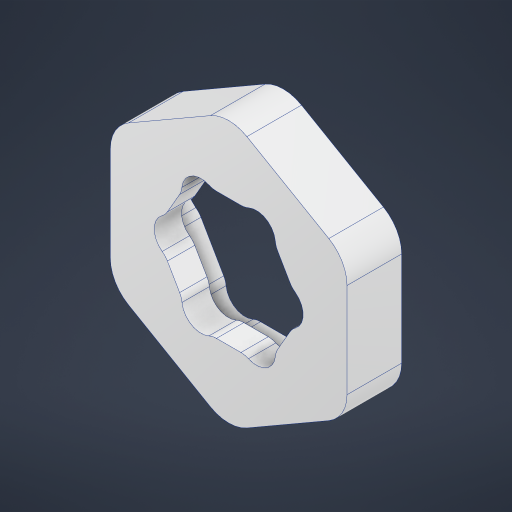
# Autodesk Inventor part: Handmade tiered cover_9mm_Wide_ALU_Cover
Saved by Autodesk Inventor 2024 (Build 280153000, 153)
## iProperties
Created: 2024-06-26
Part Number: Handmade tiered cover_9mm_Wide_ALU_Cover
Material: 알루미늄 6061
Document SubType Name: Sheet Metal
Designer: ASUS
Density: 2.7 g/cm^3
Appearance: 알루미늄 - 평지
Flat Pattern Width: 1.3 cm
Flat Pattern Length: 1.43923 cm
Flat Pattern Area: 1.871 cm^2
Sheet Metal Rule: 기본값
Sheet Metal Width: 13.000 mm
Sheet Metal Length: 14.392 mm
Sheet Metal Area: 187.100 mm^2
Author: ASUS
Autodesk Inventor part; units mm, degrees
ref_plane "YZ Plane" through (0, 0, 0) normal (1, 0, 0) x (0, 1, 0)
ref_plane "XZ Plane" through (0, 0, 0) normal (0, 1, 0) x (-1, 0, 0)
ref_plane "XY Plane" through (0, 0, 0) normal (0, 0, 1) x (1, 0, 0)
sketch "스케치1" plane through (0, 0, 0) normal (0, 0, 1) x (1, 0, 0)
  ellipse E0 centre (98.6441, 1.3888) end of major axis (99.6441, 1.3888) minor radius 1 (99.4578, 1.9701) -> (99.1441, 2.2549) ccw projected
  line L0 (99.1441, 2.2549) -> (97.9803, 2.9268) projected
  ellipse E1 centre (97.4803, 2.0608) end of major axis (98.4803, 2.0608) minor radius 1 (97.9803, 2.9268) -> (97.5768, 3.0561) ccw projected
  ellipse E2 centre (97.6782, 4.1012) end of major axis (96.6282, 4.1012) minor radius 1.05 (96.7225, 4.5359) -> (97.5768, 3.0561) ccw projected
  ellipse E3 centre (95.8122, 4.95) end of major axis (96.8122, 4.95) minor radius 1 (96.7225, 4.5359) -> (96.8122, 4.95) ccw projected
  line L1 (96.8122, 4.95) -> (96.8122, 6.2938) projected
  ellipse E4 centre (95.8122, 6.2938) end of major axis (96.8122, 6.2938) minor radius 1 (96.8122, 6.2938) -> (96.7225, 6.7079) ccw projected
  ellipse E5 centre (97.6782, 7.1426) end of major axis (96.6282, 7.1426) minor radius 1.05 (97.5768, 8.1877) -> (96.7225, 6.7079) ccw projected
  ellipse E6 centre (97.4803, 9.183) end of major axis (96.4803, 9.1831) minor radius 1 (97.5768, 8.1877) -> (97.9803, 8.317) ccw projected
  line L2 (97.9803, 8.317) -> (99.1441, 8.989) projected
  ellipse E7 centre (98.6441, 9.855) end of major axis (97.6441, 9.855) minor radius 1 (99.1441, 8.989) -> (99.4578, 9.2737) ccw projected
  ellipse E8 centre (100.3122, 8.6634) end of major axis (99.2622, 8.6634) minor radius 1.05 (101.1666, 9.2737) -> (99.4578, 9.2737) ccw projected
  ellipse E9 centre (101.9803, 9.855) end of major axis (100.9803, 9.855) minor radius 1 (101.1666, 9.2737) -> (101.4803, 8.989) ccw projected
  line L3 (101.4803, 8.989) -> (102.6441, 8.317) projected
  ellipse E10 centre (103.1441, 9.183) end of major axis (102.1441, 9.1831) minor radius 1 (102.6441, 8.317) -> (103.0476, 8.1877) ccw projected
  ellipse E11 centre (102.9462, 7.1426) end of major axis (101.8962, 7.1426) minor radius 1.05 (103.9019, 6.7079) -> (103.0476, 8.1877) ccw projected
  ellipse E12 centre (104.8122, 6.2938) end of major axis (103.8122, 6.2938) minor radius 1 (103.9019, 6.7079) -> (103.8122, 6.2938) ccw projected
  line L4 (103.8122, 6.2938) -> (103.8122, 4.95) projected
  ellipse E13 centre (104.8122, 4.95) end of major axis (103.8122, 4.95) minor radius 1 (103.8122, 4.95) -> (103.9019, 4.5359) ccw projected
  ellipse E14 centre (102.9462, 4.1012) end of major axis (101.8962, 4.1012) minor radius 1.05 (103.0476, 3.0561) -> (103.9019, 4.5359) ccw projected
  ellipse E15 centre (103.1441, 2.0608) end of major axis (104.1441, 2.0608) minor radius 1 (103.0476, 3.0561) -> (102.6441, 2.9268) ccw projected
  line L5 (102.6441, 2.9268) -> (101.4803, 2.2549) projected
  ellipse E16 centre (101.9803, 1.3888) end of major axis (102.9803, 1.3888) minor radius 1 (101.4803, 2.2549) -> (101.1666, 1.9701) ccw projected
  ellipse E17 centre (100.3122, 2.5805) end of major axis (99.2622, 2.5805) minor radius 1.05 (99.4578, 1.9701) -> (101.1666, 1.9701) ccw projected
  ellipse E18 centre (95.8122, 3.0238) end of major axis (93.8122, 3.0238) minor radius 2 (93.8122, 3.0238) -> (94.8122, 1.2918) ccw projected
  line L6 (94.8122, 1.2918) -> (99.3122, -1.3063) projected
  ellipse E19 centre (100.3122, 0.4258) end of major axis (102.3122, 0.4258) minor radius 2 (99.3122, -1.3063) -> (101.3122, -1.3063) ccw projected
  line L7 (101.3122, -1.3063) -> (105.8122, 1.2918) projected
  ellipse E20 centre (104.8122, 3.0238) end of major axis (106.8122, 3.0238) minor radius 2 (105.8122, 1.2918) -> (106.8122, 3.0238) ccw projected
  line L8 (106.8122, 3.0238) -> (106.8122, 8.22) projected
  ellipse E21 centre (104.8122, 8.22) end of major axis (106.8122, 8.22) minor radius 2 (106.8122, 8.22) -> (105.8122, 9.952) ccw projected
  line L9 (105.8122, 9.952) -> (101.3122, 12.5501) projected
  ellipse E22 centre (100.3122, 10.818) end of major axis (98.3122, 10.8181) minor radius 2 (101.3122, 12.5501) -> (99.3122, 12.5501) ccw projected
  line L10 (99.3122, 12.5501) -> (94.8122, 9.952) projected
  ellipse E23 centre (95.8122, 8.22) end of major axis (97.8122, 8.22) minor radius 2 (94.8122, 9.952) -> (93.8122, 8.22) ccw projected
  line L11 (93.8122, 8.22) -> (93.8122, 3.0238) projected
  line L12 (97.9803, 2.9239) -> (99.1441, 2.252) projected
  ellipse E24 centre (98.6441, 1.386) end of major axis (99.6441, 1.3859) minor radius 1 (99.4578, 1.9672) -> (99.1441, 2.252) ccw projected
  ellipse E25 centre (100.3122, 2.5776) end of major axis (99.2622, 2.5776) minor radius 1.05 (99.4578, 1.9672) -> (101.1666, 1.9672) ccw projected
  ellipse E26 centre (101.9803, 1.386) end of major axis (102.9803, 1.3859) minor radius 1 (101.4803, 2.252) -> (101.1666, 1.9672) ccw projected
  line L13 (101.4803, 2.252) -> (102.6441, 2.9239) projected
  ellipse E27 centre (103.1441, 2.0579) end of major axis (104.1441, 2.0579) minor radius 1 (103.0476, 3.0532) -> (102.6441, 2.9239) ccw projected
  ellipse E28 centre (102.9462, 4.0983) end of major axis (101.8962, 4.0983) minor radius 1.05 (103.0476, 3.0532) -> (103.9019, 4.533) ccw projected
  ellipse E29 centre (104.8122, 4.9471) end of major axis (105.8122, 4.9471) minor radius 1 (103.8122, 4.9471) -> (103.9019, 4.533) ccw projected
  line L14 (103.8122, 4.9471) -> (103.8122, 6.291) projected
  ellipse E30 centre (104.8122, 6.291) end of major axis (105.8122, 6.291) minor radius 1 (103.9019, 6.705) -> (103.8122, 6.291) ccw projected
  ellipse E31 centre (102.9462, 7.1397) end of major axis (101.8962, 7.1398) minor radius 1.05 (103.9019, 6.705) -> (103.0476, 8.1848) ccw projected
  ellipse E32 centre (103.1441, 9.1802) end of major axis (102.1441, 9.1802) minor radius 1 (102.6441, 8.3141) -> (103.0476, 8.1848) ccw projected
  line L15 (102.6441, 8.3141) -> (101.4803, 8.9861) projected
  ellipse E33 centre (101.9803, 9.8521) end of major axis (100.9803, 9.8521) minor radius 1 (101.1666, 9.2708) -> (101.4803, 8.9861) ccw projected
  ellipse E34 centre (100.3122, 8.6605) end of major axis (99.2622, 8.6605) minor radius 1.05 (101.1666, 9.2708) -> (99.4578, 9.2708) ccw projected
  ellipse E35 centre (98.6441, 9.8521) end of major axis (97.6441, 9.8521) minor radius 1 (99.1441, 8.9861) -> (99.4578, 9.2708) ccw projected
  line L16 (99.1441, 8.9861) -> (97.9803, 8.3141) projected
  ellipse E36 centre (97.4803, 9.1802) end of major axis (96.4803, 9.1802) minor radius 1 (97.5768, 8.1848) -> (97.9803, 8.3141) ccw projected
  ellipse E37 centre (97.6782, 7.1397) end of major axis (96.6282, 7.1398) minor radius 1.05 (97.5768, 8.1848) -> (96.7225, 6.705) ccw projected
  ellipse E38 centre (95.8122, 6.291) end of major axis (94.8122, 6.291) minor radius 1 (96.8122, 6.291) -> (96.7225, 6.705) ccw projected
  line L17 (96.8122, 6.291) -> (96.8122, 4.9471) projected
  ellipse E39 centre (95.8122, 4.9471) end of major axis (94.8122, 4.9471) minor radius 1 (96.7225, 4.533) -> (96.8122, 4.9471) ccw projected
  ellipse E40 centre (97.6782, 4.0983) end of major axis (96.6282, 4.0983) minor radius 1.05 (96.7225, 4.533) -> (97.5768, 3.0532) ccw projected
  ellipse E41 centre (97.4803, 2.0579) end of major axis (98.4803, 2.0579) minor radius 1 (97.9803, 2.9239) -> (97.5768, 3.0532) ccw projected
  ellipse E42 centre (100.3122, 5.619) end of major axis (98.1872, 5.619) minor radius 2.125 projected
  ellipse E43 centre (-1.6681, -4.2302) end of major axis (-0.6681, -4.2302) minor radius 1 (-0.8544, -3.6489) -> (-1.1681, -3.3642) ccw
  line L18 (-1.1681, -3.3642) -> (-2.3319, -2.6922)
  ellipse E44 centre (-2.8319, -3.5583) end of major axis (-1.8319, -3.5583) minor radius 1 (-2.3319, -2.6922) -> (-2.7354, -2.5629) ccw
  ellipse E45 centre (-2.634, -1.5178) end of major axis (-3.684, -1.5178) minor radius 1.05 (-3.5897, -1.0831) -> (-2.7354, -2.5629) ccw
  ellipse E46 centre (-4.5, -0.669) end of major axis (-3.5, -0.6691) minor radius 1 (-3.5897, -1.0831) -> (-3.5, -0.669) ccw
  line L19 (-3.5, -0.669) -> (-3.5, 0.6748)
  ellipse E47 centre (-4.5, 0.6748) end of major axis (-3.5, 0.6748) minor radius 1 (-3.5, 0.6748) -> (-3.5897, 1.0889) ccw
  ellipse E48 centre (-2.634, 1.5236) end of major axis (-3.684, 1.5236) minor radius 1.05 (-2.7354, 2.5687) -> (-3.5897, 1.0889) ccw
  ellipse E49 centre (-2.8319, 3.564) end of major axis (-3.8319, 3.564) minor radius 1 (-2.7354, 2.5687) -> (-2.3319, 2.698) ccw
  line L20 (-2.3319, 2.698) -> (-1.1681, 3.3699)
  ellipse E50 centre (-1.6681, 4.236) end of major axis (-2.6681, 4.236) minor radius 1 (-1.1681, 3.3699) -> (-0.8544, 3.6547) ccw
  ellipse E51 centre (0, 3.0443) end of major axis (-1.05, 3.0443) minor radius 1.05 (0.8544, 3.6547) -> (-0.8544, 3.6547) ccw
  ellipse E52 centre (1.6681, 4.236) end of major axis (0.6681, 4.236) minor radius 1 (0.8544, 3.6547) -> (1.1681, 3.3699) ccw
  line L21 (1.1681, 3.3699) -> (2.3319, 2.698)
  ellipse E53 centre (2.8319, 3.564) end of major axis (1.8319, 3.564) minor radius 1 (2.3319, 2.698) -> (2.7354, 2.5687) ccw
  ellipse E54 centre (2.634, 1.5236) end of major axis (1.584, 1.5236) minor radius 1.05 (3.5897, 1.0889) -> (2.7354, 2.5687) ccw
  ellipse E55 centre (4.5, 0.6748) end of major axis (3.5, 0.6748) minor radius 1 (3.5897, 1.0889) -> (3.5, 0.6748) ccw
  line L22 (3.5, 0.6748) -> (3.5, -0.6691)
  ellipse E56 centre (4.5, -0.6691) end of major axis (3.5, -0.669) minor radius 1 (3.5, -0.6691) -> (3.5897, -1.0831) ccw
  ellipse E57 centre (2.634, -1.5178) end of major axis (1.584, -1.5178) minor radius 1.05 (2.7354, -2.5629) -> (3.5897, -1.0831) ccw
  ellipse E58 centre (2.8319, -3.5583) end of major axis (3.8319, -3.5583) minor radius 1 (2.7354, -2.5629) -> (2.3319, -2.6922) ccw
  line L23 (2.3319, -2.6922) -> (1.1681, -3.3642)
  ellipse E59 centre (1.6681, -4.2302) end of major axis (2.6681, -4.2302) minor radius 1 (1.1681, -3.3642) -> (0.8544, -3.6489) ccw
  ellipse E60 centre (0, -3.0386) end of major axis (-1.05, -3.0386) minor radius 1.05 (-0.8544, -3.6489) -> (0.8544, -3.6489) ccw
  ellipse E61 centre (-4.5, -2.5952) end of major axis (-6.5, -2.5952) minor radius 2 (-6.5, -2.5952) -> (-5.5, -4.3272) ccw
  line L24 (-5.5, -4.3272) -> (-1, -6.9253)
  ellipse E62 centre (0, -5.1933) end of major axis (2, -5.1933) minor radius 2 (-1, -6.9253) -> (1, -6.9253) ccw
  line L25 (1, -6.9253) -> (5.5, -4.3272)
  ellipse E63 centre (4.5, -2.5952) end of major axis (6.5, -2.5952) minor radius 2 (5.5, -4.3272) -> (6.5, -2.5952) ccw
  line L26 (6.5, -2.5952) -> (6.5, 2.601)
  ellipse E64 centre (4.5, 2.601) end of major axis (6.5, 2.601) minor radius 2 (6.5, 2.601) -> (5.5, 4.333) ccw
  line L27 (5.5, 4.333) -> (1, 6.9311)
  ellipse E65 centre (0, 5.199) end of major axis (-2, 5.199) minor radius 2 (1, 6.9311) -> (-1, 6.9311) ccw
  line L28 (-1, 6.9311) -> (-5.5, 4.333)
  ellipse E66 centre (-4.5, 2.601) end of major axis (-2.5, 2.6009) minor radius 2 (-5.5, 4.333) -> (-6.5, 2.601) ccw
  line L29 (-6.5, 2.601) -> (-6.5, -2.5952)
  line L30 (-2.3319, -2.6951) -> (-1.1681, -3.367)
  ellipse E67 centre (-1.6681, -4.2331) end of major axis (-0.6681, -4.2331) minor radius 1 (-0.8544, -3.6518) -> (-1.1681, -3.367) ccw
  ellipse E68 centre (0, -3.0414) end of major axis (-1.05, -3.0414) minor radius 1.05 (-0.8544, -3.6518) -> (0.8544, -3.6518) ccw
  ellipse E69 centre (1.6681, -4.2331) end of major axis (2.6681, -4.2331) minor radius 1 (1.1681, -3.367) -> (0.8544, -3.6518) ccw
  line L31 (1.1681, -3.367) -> (2.3319, -2.6951)
  ellipse E70 centre (2.8319, -3.5611) end of major axis (3.8319, -3.5611) minor radius 1 (2.7354, -2.5658) -> (2.3319, -2.6951) ccw
  ellipse E71 centre (2.634, -1.5207) end of major axis (1.584, -1.5207) minor radius 1.05 (2.7354, -2.5658) -> (3.5897, -1.086) ccw
  ellipse E72 centre (4.5, -0.6719) end of major axis (5.5, -0.6719) minor radius 1 (3.5, -0.6719) -> (3.5897, -1.086) ccw
  line L32 (3.5, -0.6719) -> (3.5, 0.6719)
  ellipse E73 centre (4.5, 0.6719) end of major axis (5.5, 0.6719) minor radius 1 (3.5897, 1.086) -> (3.5, 0.6719) ccw
  ellipse E74 centre (2.634, 1.5207) end of major axis (1.584, 1.5207) minor radius 1.05 (3.5897, 1.086) -> (2.7354, 2.5658) ccw
  ellipse E75 centre (2.8319, 3.5611) end of major axis (1.8319, 3.5611) minor radius 1 (2.3319, 2.6951) -> (2.7354, 2.5658) ccw
  line L33 (2.3319, 2.6951) -> (1.1681, 3.367)
  ellipse E76 centre (1.6681, 4.2331) end of major axis (0.6681, 4.2331) minor radius 1 (0.8544, 3.6518) -> (1.1681, 3.367) ccw
  ellipse E77 centre (0, 3.0414) end of major axis (-1.05, 3.0415) minor radius 1.05 (0.8544, 3.6518) -> (-0.8544, 3.6518) ccw
  ellipse E78 centre (-1.6681, 4.2331) end of major axis (-2.6681, 4.2331) minor radius 1 (-1.1681, 3.367) -> (-0.8544, 3.6518) ccw
  line L34 (-1.1681, 3.367) -> (-2.3319, 2.6951)
  ellipse E79 centre (-2.8319, 3.5611) end of major axis (-3.8319, 3.5611) minor radius 1 (-2.7354, 2.5658) -> (-2.3319, 2.6951) ccw
  ellipse E80 centre (-2.634, 1.5207) end of major axis (-3.684, 1.5207) minor radius 1.05 (-2.7354, 2.5658) -> (-3.5897, 1.086) ccw
  ellipse E81 centre (-4.5, 0.6719) end of major axis (-5.5, 0.6719) minor radius 1 (-3.5, 0.6719) -> (-3.5897, 1.086) ccw
  line L35 (-3.5, 0.6719) -> (-3.5, -0.6719)
  ellipse E82 centre (-4.5, -0.6719) end of major axis (-5.5, -0.6719) minor radius 1 (-3.5897, -1.086) -> (-3.5, -0.6719) ccw
  ellipse E83 centre (-2.634, -1.5207) end of major axis (-3.684, -1.5207) minor radius 1.05 (-3.5897, -1.086) -> (-2.7354, -2.5658) ccw
  ellipse E84 centre (-2.8319, -3.5611) end of major axis (-1.8319, -3.5611) minor radius 1 (-2.3319, -2.6951) -> (-2.7354, -2.5658) ccw
  ellipse E85 centre (0, 0) end of major axis (-2.125, 0) minor radius 2.125
  point P0 (-3.684, -1.5193)
  point P1 (-3.684, 1.5222)
  point P2 (3.684, 1.5222)
  point P3 (3.5, 0.6721)
  point P4 (3.684, -1.5193)
  constraints: 36 end point, 213 other
extrude "돌출1" add sketch "스케치1" along normal blind 3 contours L29 E66 L28 E65 L27 E64 L26 E63 L25 E62 L24 E61
sketch "스케치2" plane through (0, 0, 3) normal (0, 0, 1) x (1, 0, 0)
  ellipse E0 centre (-4.5, -2.5952) end of major axis (-6.5, -2.5952) minor radius 2 (-6.5, -2.5952) -> (-5.5, -4.3272) ccw projected
  line L0 (-5.5, -4.3272) -> (-1, -6.9253) projected
  ellipse E1 centre (0, -5.1933) end of major axis (2, -5.1933) minor radius 2 (-1, -6.9253) -> (1, -6.9253) ccw projected
  line L1 (1, -6.9253) -> (5.5, -4.3272) projected
  ellipse E2 centre (4.5, -2.5952) end of major axis (6.5, -2.5952) minor radius 2 (5.5, -4.3272) -> (6.5, -2.5952) ccw projected
  line L2 (6.5, -2.5952) -> (6.5, 2.601) projected
  ellipse E3 centre (4.5, 2.601) end of major axis (6.5, 2.601) minor radius 2 (6.5, 2.601) -> (5.5, 4.333) ccw projected
  line L3 (5.5, 4.333) -> (1, 6.9311) projected
  ellipse E4 centre (0, 5.199) end of major axis (-2, 5.199) minor radius 2 (1, 6.9311) -> (-1, 6.9311) ccw projected
  line L4 (-1, 6.9311) -> (-5.5, 4.333) projected
  ellipse E5 centre (-4.5, 2.601) end of major axis (-2.5, 2.6009) minor radius 2 (-5.5, 4.333) -> (-6.5, 2.601) ccw projected
  line L5 (-6.5, 2.601) -> (-6.5, -2.5952) projected
  ellipse E6 centre (-2.8319, -3.5611) end of major axis (-1.8319, -3.5611) minor radius 1 (-2.3319, -2.6951) -> (-2.7354, -2.5658) ccw projected
  ellipse E7 centre (-2.634, -1.5207) end of major axis (-1.584, -1.5207) minor radius 1.05 (-3.684, -1.5193) -> (-2.7354, -2.5658) ccw projected
  ellipse E8 centre (-2.634, -1.5178) end of major axis (-1.584, -1.5178) minor radius 1.05 (-3.5897, -1.0831) -> (-3.684, -1.5193) ccw projected
  ellipse E9 centre (-4.5, -0.669) end of major axis (-3.5, -0.6691) minor radius 1 (-3.5897, -1.0831) -> (-3.5, -0.669) ccw projected
  line L6 (-3.5, -0.669) -> (-3.5, 0.6748) projected
  ellipse E10 centre (-4.5, 0.6719) end of major axis (-5.5, 0.6719) minor radius 1 (-3.5, 0.6748) -> (-3.5897, 1.086) ccw projected
  ellipse E11 centre (-2.634, 1.5207) end of major axis (-1.584, 1.5207) minor radius 1.05 (-3.684, 1.5222) -> (-3.5897, 1.086) ccw projected
  ellipse E12 centre (-2.634, 1.5236) end of major axis (-1.584, 1.5236) minor radius 1.05 (-2.7354, 2.5687) -> (-3.684, 1.5222) ccw projected
  ellipse E13 centre (-2.8319, 3.564) end of major axis (-3.8319, 3.564) minor radius 1 (-2.7354, 2.5687) -> (-2.3319, 2.698) ccw projected
  line L7 (-2.3319, 2.698) -> (-1.1681, 3.3699) projected
  ellipse E14 centre (-1.6681, 4.236) end of major axis (-2.6681, 4.236) minor radius 1 (-1.1681, 3.3699) -> (-0.8544, 3.6547) ccw projected
  ellipse E15 centre (0, 3.0443) end of major axis (1.05, 3.0443) minor radius 1.05 (0.8544, 3.6547) -> (-0.8544, 3.6547) ccw projected
  ellipse E16 centre (1.6681, 4.236) end of major axis (0.6681, 4.236) minor radius 1 (0.8544, 3.6547) -> (1.1681, 3.3699) ccw projected
  line L8 (1.1681, 3.3699) -> (2.3319, 2.698) projected
  ellipse E17 centre (2.8319, 3.564) end of major axis (1.8319, 3.564) minor radius 1 (2.3319, 2.698) -> (2.7354, 2.5687) ccw projected
  ellipse E18 centre (2.634, 1.5236) end of major axis (3.684, 1.5236) minor radius 1.05 (3.684, 1.5222) -> (2.7354, 2.5687) ccw projected
  ellipse E19 centre (2.634, 1.5207) end of major axis (3.684, 1.5207) minor radius 1.05 (3.5897, 1.086) -> (3.684, 1.5222) ccw projected
  ellipse E20 centre (4.5, 0.6719) end of major axis (5.5, 0.6719) minor radius 1 (3.5897, 1.086) -> (3.5, 0.6721) ccw projected
  line L9 (3.5, 0.6721) -> (3.5, -0.6691) projected
  ellipse E21 centre (4.5, -0.6691) end of major axis (3.5, -0.669) minor radius 1 (3.5, -0.6691) -> (3.5897, -1.0831) ccw projected
  ellipse E22 centre (2.634, -1.5178) end of major axis (3.684, -1.5178) minor radius 1.05 (3.684, -1.5193) -> (3.5897, -1.0831) ccw projected
  ellipse E23 centre (2.634, -1.5207) end of major axis (3.684, -1.5207) minor radius 1.05 (2.7354, -2.5658) -> (3.684, -1.5193) ccw projected
  ellipse E24 centre (2.8319, -3.5611) end of major axis (3.8319, -3.5611) minor radius 1 (2.7354, -2.5658) -> (2.3319, -2.6951) ccw projected
  line L10 (2.3319, -2.6951) -> (1.1681, -3.367) projected
  ellipse E25 centre (1.6681, -4.2331) end of major axis (2.6681, -4.2331) minor radius 1 (1.1681, -3.367) -> (0.8544, -3.6518) ccw projected
  ellipse E26 centre (0, -3.0414) end of major axis (1.05, -3.0415) minor radius 1.05 (-0.8544, -3.6518) -> (0.8544, -3.6518) ccw projected
  ellipse E27 centre (-1.6681, -4.2331) end of major axis (-0.6681, -4.2331) minor radius 1 (-0.8544, -3.6518) -> (-1.1681, -3.367) ccw projected
  line L11 (-1.1681, -3.367) -> (-2.3319, -2.6951) projected
  point P0 (0, 0)
  constraints: 28 other
extrude "돌출2" add sketch "스케치2" against normal up to surface (3 mm away) contours E6 E7 E8 E9 L6 E10 E11 E12 E13 L7 E14 E15 E16 L8 E17 E18 E19 E20 L9 E21 E22 E23 E24 L10 E25 E26 E27 L11
sketch "스케치3" plane through (0, 0, 3) normal (0, 0, 1) x (1, 0, 0)
  ellipse E0 centre (-4.5, -2.5952) end of major axis (-6.5, -2.5952) minor radius 2 (-6.5, -2.5952) -> (-5.5, -4.3272) ccw projected
  line L0 (-5.5, -4.3272) -> (-1, -6.9253) projected
  ellipse E1 centre (0, -5.1933) end of major axis (2, -5.1933) minor radius 2 (-1, -6.9253) -> (1, -6.9253) ccw projected
  line L1 (1, -6.9253) -> (5.5, -4.3272) projected
  ellipse E2 centre (4.5, -2.5952) end of major axis (6.5, -2.5952) minor radius 2 (5.5, -4.3272) -> (6.5, -2.5952) ccw projected
  line L2 (6.5, -2.5952) -> (6.5, 2.601) projected
  ellipse E3 centre (4.5, 2.601) end of major axis (6.5, 2.601) minor radius 2 (6.5, 2.601) -> (5.5, 4.333) ccw projected
  line L3 (5.5, 4.333) -> (1, 6.9311) projected
  ellipse E4 centre (0, 5.199) end of major axis (-2, 5.199) minor radius 2 (1, 6.9311) -> (-1, 6.9311) ccw projected
  line L4 (-1, 6.9311) -> (-5.5, 4.333) projected
  ellipse E5 centre (-4.5, 2.601) end of major axis (-2.5, 2.6009) minor radius 2 (-5.5, 4.333) -> (-6.5, 2.601) ccw projected
  line L5 (-6.5, 2.601) -> (-6.5, -2.5952) projected
  line L6 (4.0415, 0.002) -> (2.0225, -3.499)
  line L7 (2.0225, -3.499) -> (-2.019, -3.501)
  line L8 (-2.019, -3.501) -> (-4.0415, -0.002)
  line L9 (-4.0415, -0.002) -> (-2.0225, 3.499)
  line L10 (-2.0225, 3.499) -> (2.019, 3.501)
  line L11 (2.019, 3.501) -> (4.0415, 0.002)
  line L12 (2.019, 3.501) -> (1.519, 2.635)
  line L13 (2.019, 3.501) -> (3.019, 3.501) construction
  circle A0 centre (1.519, 2.635) radius 1.05
  circle A1 centre (-1.5225, 2.633) radius 1.05
  circle A2 centre (-3.0415, -0.002) radius 1.05
  circle A3 centre (-1.519, -2.635) radius 1.05
  circle A4 centre (1.5225, -2.633) radius 1.05
  circle A5 centre (3.0415, 0.002) radius 1.05
  point P0 (0, 0)
  point P1 (0, 0)
  point P2 (0.9245, 3.5005)
  point P3 (-0.9295, 3.4995)
  point P4 (-2.5692, 2.5509)
  point P5 (-3.4955, 0.9448)
  point P6 (-3.4937, -0.9496)
  point P7 (-2.5659, -2.5548)
  point P8 (-0.9245, -3.5005)
  point P9 (0.9295, -3.4995)
  point P10 (2.5692, -2.5509)
  point P11 (3.4955, -0.9448)
  point P12 (3.4937, 0.9496)
  point P13 (2.5659, 2.5548)
  dimension "d4" = 7
  dimension "d5" = 1
  dimension "d6" = 120
  dimension "d7" = 2.1
  dimension "d10" = 360
  constraints: 16 end point, 6 centre point, 2 coincident, 1 equal length, 1 horizontal, 32 other
  measures "d4" distance between parallel lines of L8 L11
  measures "d5" distance of L10.end L12.end
  measures "d6" angle of L12 L13
  measures "d7" diameter of A0
extrude "돌출3" cut sketch "스케치3" against normal blind 1.5 contours L11 A5 L6 | L6 A5 L11 | L6 A4 L7 A3 L8 A2 L9 A1 L10 A0 L11 A5 | A4 L7 L6 | L6 L7 A4 | A0 L10 L11 | L11 L10 A0 | A3 L8 L7 | L7 L8 A3 | A1 L9 L10 | L10 L9 A1 | A2 L9 L8 | L8 L9 A2
sketch "스케치4" plane through (0, 0, 1.5) normal (0, 0, 1) x (1, 0, 0)
  arc A0 (-0.9295, 3.4995) -> (-2.5692, 2.5509) centre (-1.5225, 2.633) ccw projected
  line L0 (-3.4955, 0.9448) -> (-2.5692, 2.5509) projected
  arc A1 (-3.4955, 0.9448) -> (-3.4937, -0.9496) centre (-3.0415, -0.002) ccw projected
  line L1 (-2.5659, -2.5548) -> (-3.4937, -0.9496) projected
  arc A2 (-2.5659, -2.5548) -> (-0.9245, -3.5005) centre (-1.519, -2.635) ccw projected
  line L2 (0.9295, -3.4995) -> (-0.9245, -3.5005) projected
  arc A3 (0.9295, -3.4995) -> (2.5692, -2.5509) centre (1.5225, -2.633) ccw projected
  line L3 (3.4955, -0.9448) -> (2.5692, -2.5509) projected
  arc A4 (3.4955, -0.9448) -> (3.4937, 0.9496) centre (3.0415, 0.002) ccw projected
  line L4 (2.5659, 2.5548) -> (3.4937, 0.9496) projected
  arc A5 (2.5659, 2.5548) -> (0.9245, 3.5005) centre (1.519, 2.635) ccw projected
  line L5 (-0.9295, 3.4995) -> (0.9245, 3.5005) projected
  circle A6 centre (0, 0) radius 2
  dimension "d14" = 4
  constraints: 1 centre point, 1 coincident
  measures "d14" diameter of A6
extrude "돌출4" cut sketch "스케치4" against normal through all contours A6
fillet "모깎기1" radius 1 2 edges at (2.5659, 2.5548, 2.25) (3.4937, 0.9496, 2.25)
pattern_circular "원형 패턴1" count 6 over 360 about axis through (0, 0, 1.5) along (0, 0, -1) of "모깎기1", "돌출4"
sketch "스케치5" plane through (0, 0, 1.5) normal (0, 0, 1) x (1, 0, 0)
  circle A0 centre (0, 0) radius 2 projected
  line L0 (-3.3681, 1.1656) -> (-2.6968, 2.3297) projected
  arc A1 (-3.6525, 0.8519) -> (-3.3681, 1.1656) centre (-4.2344, 1.6652) ccw projected
  arc A2 (-3.6525, 0.8519) -> (-3.6511, -0.8569) centre (-3.0415, -0.002) ccw projected
  arc A3 (-3.366, -1.1706) -> (-3.6511, -0.8569) centre (-4.2318, -1.671) ccw projected
  line L1 (-2.6935, -2.3341) -> (-3.366, -1.1706) projected
  arc A4 (-2.564, -2.7372) -> (-2.6935, -2.3341) centre (-3.5593, -2.8345) ccw projected
  arc A5 (-2.564, -2.7372) -> (-1.0835, -3.5904) centre (-1.519, -2.635) ccw projected
  arc A6 (-0.6692, -3.5003) -> (-1.0835, -3.5904) centre (-0.6687, -4.5003) ccw projected
  line L2 (0.6746, -3.4997) -> (-0.6692, -3.5003) projected
  arc A7 (1.0885, -3.5891) -> (0.6746, -3.4997) centre (0.6751, -4.4997) ccw projected
  arc A8 (1.0885, -3.5891) -> (2.5676, -2.7335) centre (1.5225, -2.633) ccw projected
  arc A9 (2.6968, -2.3297) -> (2.5676, -2.7335) centre (3.563, -2.8293) ccw projected
  line L3 (3.3681, -1.1656) -> (2.6968, -2.3297) projected
  arc A10 (3.6525, -0.8519) -> (3.3681, -1.1656) centre (4.2344, -1.6652) ccw projected
  arc A11 (3.6525, -0.8519) -> (3.6511, 0.8569) centre (3.0415, 0.002) ccw projected
  arc A12 (3.366, 1.1706) -> (3.6511, 0.8569) centre (4.2318, 1.671) ccw projected
  line L4 (2.6935, 2.3341) -> (3.366, 1.1706) projected
  arc A13 (2.564, 2.7372) -> (2.6935, 2.3341) centre (3.5593, 2.8345) ccw projected
  arc A14 (2.564, 2.7372) -> (1.0835, 3.5904) centre (1.519, 2.635) ccw projected
  arc A15 (0.6692, 3.5003) -> (1.0835, 3.5904) centre (0.6687, 4.5003) ccw projected
  line L5 (-0.6746, 3.4997) -> (0.6692, 3.5003) projected
  arc A16 (-1.0885, 3.5891) -> (-0.6746, 3.4997) centre (-0.6751, 4.4997) ccw projected
  arc A17 (-1.0885, 3.5891) -> (-2.5676, 2.7335) centre (-1.5225, 2.633) ccw projected
  arc A18 (-2.6968, 2.3297) -> (-2.5676, 2.7335) centre (-3.563, 2.8293) ccw projected
  circle A19 centre (0, 0) radius 2.5
  dimension "d21" = 5
  constraints: 1 centre point, 1 coincident
  measures "d21" diameter of A19
extrude "돌출5" cut sketch "스케치5" against normal through all contours A0 | A19
sketch "스케치6" plane through (0, 0, 0) normal (0, 0, -1) x (-1, 0, 0)
  circle A0 centre (0, 0) radius 2.5 projected
  ellipse E0 centre (4.5, -2.5952) end of major axis (6.5, -2.5952) minor radius 2 (5.5, -4.3272) -> (6.5, -2.5952) ccw projected
  line L0 (6.5, 2.601) -> (6.5, -2.5952) projected
  ellipse E1 centre (4.5, 2.601) end of major axis (2.5, 2.6009) minor radius 2 (6.5, 2.601) -> (5.5, 4.333) ccw projected
  line L1 (1, 6.9311) -> (5.5, 4.333) projected
  ellipse E2 centre (0, 5.199) end of major axis (2, 5.199) minor radius 2 (1, 6.9311) -> (-1, 6.9311) ccw projected
  line L2 (-5.5, 4.333) -> (-1, 6.9311) projected
  ellipse E3 centre (-4.5, 2.601) end of major axis (-6.5, 2.601) minor radius 2 (-5.5, 4.333) -> (-6.5, 2.601) ccw projected
  line L3 (-6.5, -2.5952) -> (-6.5, 2.601) projected
  ellipse E4 centre (-4.5, -2.5952) end of major axis (-6.5, -2.5952) minor radius 2 (-6.5, -2.5952) -> (-5.5, -4.3272) ccw projected
  line L4 (-1, -6.9253) -> (-5.5, -4.3272) projected
  ellipse E5 centre (0, -5.1933) end of major axis (-2, -5.1933) minor radius 2 (-1, -6.9253) -> (1, -6.9253) ccw projected
  line L5 (5.5, -4.3272) -> (1, -6.9253) projected
  line L6 (5.1962, 0.0025) -> (2.6002, -4.4988)
  line L7 (2.6002, -4.4988) -> (-2.5959, -4.5012)
  line L8 (-2.5959, -4.5012) -> (-5.1962, -0.0025)
  line L9 (-5.1962, -0.0025) -> (-2.6002, 4.4988)
  line L10 (-2.6002, 4.4988) -> (2.5959, 4.5012)
  line L11 (2.5959, 4.5012) -> (5.1962, 0.0025)
  dimension "d24" = 9
  constraints: 12 end point, 1 coincident, 19 other
  measures "d24" distance between parallel lines of L8 L11
extrude "돌출6" cut sketch "스케치6" against normal blind 1.5 contours L6 L7 L8 L9 L10 L11
sketch "스케치7" plane through (0, 0, 0) normal (0, 0, -1) x (-1, 0, 0)
  line L0 (-5.1962, -0.0025) -> (-2.6002, 4.4988) projected
  line L1 (-2.6002, 4.4988) -> (2.5959, 4.5012) projected
  line L2 (2.5959, 4.5012) -> (5.1962, 0.0025) projected
  line L3 (5.1962, 0.0025) -> (2.6002, -4.4988) projected
  line L4 (2.6002, -4.4988) -> (-2.5959, -4.5012) projected
  line L5 (-2.5959, -4.5012) -> (-5.1962, -0.0025) projected
  ellipse E0 centre (4.5, -2.5952) end of major axis (6.5, -2.5952) minor radius 2 (5.5, -4.3272) -> (6.5, -2.5952) ccw projected
  line L6 (6.5, 2.601) -> (6.5, -2.5952) projected
  ellipse E1 centre (4.5, 2.601) end of major axis (2.5, 2.6009) minor radius 2 (6.5, 2.601) -> (5.5, 4.333) ccw projected
  line L7 (1, 6.9311) -> (5.5, 4.333) projected
  ellipse E2 centre (0, 5.199) end of major axis (2, 5.199) minor radius 2 (1, 6.9311) -> (-1, 6.9311) ccw projected
  line L8 (-5.5, 4.333) -> (-1, 6.9311) projected
  ellipse E3 centre (-4.5, 2.601) end of major axis (-6.5, 2.601) minor radius 2 (-5.5, 4.333) -> (-6.5, 2.601) ccw projected
  line L9 (-6.5, -2.5952) -> (-6.5, 2.601) projected
  ellipse E4 centre (-4.5, -2.5952) end of major axis (-6.5, -2.5952) minor radius 2 (-6.5, -2.5952) -> (-5.5, -4.3272) ccw projected
  line L10 (-1, -6.9253) -> (-5.5, -4.3272) projected
  ellipse E5 centre (0, -5.1933) end of major axis (-2, -5.1933) minor radius 2 (-1, -6.9253) -> (1, -6.9253) ccw projected
  line L11 (5.5, -4.3272) -> (1, -6.9253) projected
  line L12 (5.1962, 0.0025) -> (4.1962, 0.0025)
  circle A0 centre (4.1962, 0.0025) radius 1.05
  circle A1 centre (2.0959, 3.6352) radius 1.05
  circle A2 centre (-2.1002, 3.6327) radius 1.05
  circle A3 centre (-4.1962, -0.0025) radius 1.05
  circle A4 centre (-2.0959, -3.6352) radius 1.05
  circle A5 centre (2.1002, -3.6327) radius 1.05
  point P0 (0, 0)
  dimension "d27" = 1
  dimension "d28" = 2.1
  dimension "d33" = 360
  constraints: 6 centre point, 2 end point, 1 coincident, 1 horizontal, 19 other
  measures "d27" distance of L2.end L12.end
  measures "d28" diameter of A0
extrude "돌출7" cut sketch "스케치7" against normal blind 1.5 contours L5 A3 L0 | L0 A3 L5 | A2 L1 L0 | L0 L1 A2 | A4 L4 L5 | L5 L4 A4 | A1 L2 L1 | L1 L2 A1 | A5 L3 L4 | L4 L3 A5 | A0 L3 L2 | L2 L3 A0
fillet "모깎기2" radius 1 12 edges at (-4.6501, -0.9443, 0.75) (-4.6485, 0.9501, 0.75) (-3.147, -3.5507, 0.75) (-1.5073, -4.4993, 0.75) (1.5015, -4.5007, 0.75) (3.1429, -3.555, 0.75) (4.6485, -0.9501, 0.75) (4.6501, 0.9443, 0.75) (3.147, 3.5507, 0.75) (1.5073, 4.4993, 0.75) (-3.1429, 3.555, 0.75) (-1.5015, 4.5007, 0.75)
equation "\"TransitionRadius\" = BendRadius"
equation "\"BendRadius\" = 3.048"
